nail_polish (Autodesk Fusion 360 design; units mm, degrees)
Autodesk Fusion 360 part; units mm, degrees
sketch "Sketch1" plane through (0, 0, 0) normal (0, 0, 1) x (1, 0, 0)
  line L0 (0, 0) -> (-170, 0)
  line L1 (-170, 0) -> (-170, 170)
  line L2 (-170, 170) -> (0, 170)
  line L3 (0, 170) -> (0, 0)
  line L4 (-5, 5) -> (-33.5, 5)
  line L5 (-33.5, 5) -> (-33.5, 33.5)
  line L6 (-33.5, 33.5) -> (-5, 33.5)
  line L7 (-5, 33.5) -> (-5, 5)
  dimension "d1" = 170
  dimension "d2" = 28.5
  dimension "d3" = 28.5
  dimension "d4" = 5
  dimension "d5" = 5
  dimension "d8" = 170
  constraint horizontal L0
  constraint vertical L1
  constraint horizontal L2
  constraint vertical L3
  constraint coincident L0.start L3.end
  constraint horizontal L4
  constraint vertical L5
  constraint horizontal L6
  constraint vertical L7
  measures "d1" distance of L1.end L2.end
  measures "d2" distance of L4.start L6.end
  measures "d3" distance of L4.start L4.end
  measures "d4" distance of L0 L4
  measures "d5" distance of L3 L7
  measures "d8" distance of L0.end L1.end
extrude "Extrude1" add sketch "Sketch1" along normal blind 13 contours L0 L1 L2 L3 | L4 L5 L6 L7
extrude "Extrude2" cut sketch "Sketch1" along normal blind 8 contours L4 L5 L6 L7
pattern_linear "R-Pattern1" count 5 spacing 32.875 along (-1, 0, 0) count 5 spacing 32.875 along (0, 1, 0) of "Extrude2"
chamfer "Chamfer1" distance 2 distance2 8 100 edges at (-19.25, 33.5, 0) (-19.25, 66.375, 0) (-19.25, 99.25, 0) (-19.25, 132.125, 0) (-19.25, 165, 0) (-52.125, 165, 0) (-85, 165, 0) (-117.875, 165, 0) (-150.75, 165, 0) (-150.75, 132.125, 0) (-117.875, 132.125, 0) (-85, 132.125, 0) (-52.125, 132.125, 0) (-52.125, 99.25, 0) (-85, 99.25, 0) (-117.875, 99.25, 0) (-150.75, 99.25, 0) (-150.75, 66.375, 0) (-117.875, 66.375, 0) (-132.125, 85, 0) (-103.625, 85, 0) (-99.25, 85, 0) (-70.75, 85, 0) (-66.375, 85, 0) (-37.875, 85, 0) (-33.5, 85, 0) (-5, 85, 0) (-52.125, 66.375, 0) (-52.125, 33.5, 0) (-85, 33.5, 0) (-117.875, 33.5, 0) (-150.75, 33.5, 0) (-85, 66.375, 0) (-5, 150.75, 0) (-33.5, 150.75, 0) (-37.875, 150.75, 0) (-66.375, 150.75, 0) (-70.75, 150.75, 0) (-99.25, 150.75, 0) (-103.625, 150.75, 0) (-132.125, 150.75, 0) (-136.5, 150.75, 0) (-165, 150.75, 0) (-165, 117.875, 0) (-136.5, 117.875, 0) (-132.125, 117.875, 0) (-103.625, 117.875, 0) (-99.25, 117.875, 0) (-70.75, 117.875, 0) (-66.375, 117.875, 0) (-37.875, 117.875, 0) (-33.5, 117.875, 0) (-5, 117.875, 0) (-19.25, 70.75, 0) (-52.125, 70.75, 0) (-85, 70.75, 0) (-117.875, 70.75, 0) (-150.75, 70.75, 0) (-136.5, 85, 0) (-165, 85, 0) (-165, 52.125, 0) (-136.5, 52.125, 0) (-132.125, 52.125, 0) (-103.625, 52.125, 0) (-99.25, 52.125, 0) (-70.75, 52.125, 0) (-66.375, 52.125, 0) (-37.875, 52.125, 0) (-33.5, 52.125, 0) (-5, 52.125, 0) (-19.25, 37.875, 0) (-52.125, 37.875, 0) (-85, 37.875, 0) (-117.875, 37.875, 0) (-150.75, 37.875, 0) (-165, 19.25, 0) (-136.5, 19.25, 0) (-132.125, 19.25, 0) (-103.625, 19.25, 0) (-99.25, 19.25, 0) (-70.75, 19.25, 0) (-66.375, 19.25, 0) (-37.875, 19.25, 0) (-33.5, 19.25, 0) (-5, 19.25, 0) (-19.25, 5, 0) (-52.125, 5, 0) (-85, 5, 0) (-117.875, 5, 0) (-150.75, 5, 0) (-150.75, 103.625, 0) (-117.875, 103.625, 0) (-85, 103.625, 0) (-52.125, 103.625, 0) (-19.25, 103.625, 0) (-19.25, 136.5, 0) (-52.125, 136.5, 0) (-85, 136.5, 0) (-117.875, 136.5, 0) (-150.75, 136.5, 0) measured on face at (-80.25, 1.6667, 0) measured on face at (-80.25, 1.6667, 0) measured on face at (-80.25, 1.6667, 0) measured on face at (-80.25, 1.6667, 0) measured on face at (-80.25, 1.6667, 0) measured on face at (-80.25, 1.6667, 0) measured on face at (-80.25, 1.6667, 0) measured on face at (-80.25, 1.6667, 0) measured on face at (-80.25, 1.6667, 0) measured on face at (-80.25, 1.6667, 0) measured on face at (-80.25, 1.6667, 0) measured on face at (-80.25, 1.6667, 0) measured on face at (-80.25, 1.6667, 0) measured on face at (-80.25, 1.6667, 0) measured on face at (-80.25, 1.6667, 0) measured on face at (-80.25, 1.6667, 0) measured on face at (-80.25, 1.6667, 0) measured on face at (-80.25, 1.6667, 0) measured on face at (-80.25, 1.6667, 0) measured on face at (-80.25, 1.6667, 0) measured on face at (-80.25, 1.6667, 0) measured on face at (-80.25, 1.6667, 0) measured on face at (-80.25, 1.6667, 0) measured on face at (-80.25, 1.6667, 0) measured on face at (-80.25, 1.6667, 0) measured on face at (-80.25, 1.6667, 0) measured on face at (-80.25, 1.6667, 0) measured on face at (-80.25, 1.6667, 0) measured on face at (-80.25, 1.6667, 0) measured on face at (-80.25, 1.6667, 0) measured on face at (-80.25, 1.6667, 0) measured on face at (-80.25, 1.6667, 0) measured on face at (-80.25, 1.6667, 0) measured on face at (-80.25, 1.6667, 0) measured on face at (-80.25, 1.6667, 0) measured on face at (-80.25, 1.6667, 0) measured on face at (-80.25, 1.6667, 0) measured on face at (-80.25, 1.6667, 0) measured on face at (-80.25, 1.6667, 0) measured on face at (-80.25, 1.6667, 0) measured on face at (-80.25, 1.6667, 0) measured on face at (-80.25, 1.6667, 0) measured on face at (-80.25, 1.6667, 0) measured on face at (-80.25, 1.6667, 0) measured on face at (-80.25, 1.6667, 0) measured on face at (-80.25, 1.6667, 0) measured on face at (-80.25, 1.6667, 0) measured on face at (-80.25, 1.6667, 0) measured on face at (-80.25, 1.6667, 0) measured on face at (-80.25, 1.6667, 0) measured on face at (-80.25, 1.6667, 0) measured on face at (-80.25, 1.6667, 0) measured on face at (-80.25, 1.6667, 0) measured on face at (-80.25, 1.6667, 0) measured on face at (-80.25, 1.6667, 0) measured on face at (-80.25, 1.6667, 0) measured on face at (-80.25, 1.6667, 0) measured on face at (-80.25, 1.6667, 0) measured on face at (-80.25, 1.6667, 0) measured on face at (-80.25, 1.6667, 0) measured on face at (-80.25, 1.6667, 0) measured on face at (-80.25, 1.6667, 0) measured on face at (-80.25, 1.6667, 0) measured on face at (-80.25, 1.6667, 0) measured on face at (-80.25, 1.6667, 0) measured on face at (-80.25, 1.6667, 0) measured on face at (-80.25, 1.6667, 0) measured on face at (-80.25, 1.6667, 0) measured on face at (-80.25, 1.6667, 0) measured on face at (-80.25, 1.6667, 0) measured on face at (-80.25, 1.6667, 0) measured on face at (-80.25, 1.6667, 0) measured on face at (-80.25, 1.6667, 0) measured on face at (-80.25, 1.6667, 0) measured on face at (-80.25, 1.6667, 0) measured on face at (-80.25, 1.6667, 0) measured on face at (-80.25, 1.6667, 0) measured on face at (-80.25, 1.6667, 0) measured on face at (-80.25, 1.6667, 0) measured on face at (-80.25, 1.6667, 0) measured on face at (-80.25, 1.6667, 0) measured on face at (-80.25, 1.6667, 0) measured on face at (-80.25, 1.6667, 0) measured on face at (-80.25, 1.6667, 0) measured on face at (-80.25, 1.6667, 0) measured on face at (-80.25, 1.6667, 0) measured on face at (-80.25, 1.6667, 0) measured on face at (-80.25, 1.6667, 0) measured on face at (-80.25, 1.6667, 0) measured on face at (-80.25, 1.6667, 0) measured on face at (-80.25, 1.6667, 0) measured on face at (-80.25, 1.6667, 0) measured on face at (-80.25, 1.6667, 0) measured on face at (-80.25, 1.6667, 0) measured on face at (-80.25, 1.6667, 0) measured on face at (-80.25, 1.6667, 0) measured on face at (-80.25, 1.6667, 0) measured on face at (-80.25, 1.6667, 0) measured on face at (-80.25, 1.6667, 0) measured on face at (-80.25, 1.6667, 0)
equation "d1 = ( 340 / 2 ) * 1 mm"
equation "d3 = d2"
equation "d5 = d4"
equation "d8 = d1"
